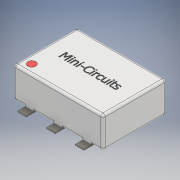
# Autodesk Inventor part: Transformer_CD542
Saved by Autodesk Inventor 2018 (Build 220112000, 112)
## iProperties
Created: 2019-01-11
Part Number: Transformer_CD542
Material: Copper
Document SubType Name: Modeling
Designer: Bradley
Density: 8.94 g/cm^3
Appearance: Smooth - White
Author: Bradley
Autodesk Inventor part; units mm, degrees
ref_plane "YZ Plane" through (0, 0, 0) normal (1, 0, 0) x (0, 1, 0)
ref_plane "XZ Plane" through (0, 0, 0) normal (0, 1, 0) x (-1, 0, 0)
ref_plane "XY Plane" through (0, 0, 0) normal (0, 0, 1) x (1, 0, 0)
sketch "Sketch1" plane through (0, 0, 0) normal (0, 0, 1) x (1, 0, 0)
  line L0 (-3.935, -2.795) -> (3.935, -2.795)
  line L1 (3.935, -2.795) -> (3.935, 2.795)
  line L2 (3.935, 2.795) -> (-3.935, 2.795)
  line L3 (-3.935, 2.795) -> (-3.935, -2.795)
  line L4 (-3.935, -2.795) -> (3.935, 2.795) construction
  line L5 (3.935, -2.795) -> (-3.935, 2.795) construction
  point P0 (0, 0)
  dimension "d0" = 7.87
  dimension "d1" = 5.59
  constraints: 12 end point, 2 midpoint, 2 parallel, 1 horizontal, 1 perpendicular
  measures "d0" distance of L2.end L1.end
  measures "d1" distance of L1.end L0.end
extrude "Extrusion1" add sketch "Sketch1" along normal blind 2.74
sketch "Sketch2" plane through (0, 0, 0) normal (0, 0, -1) x (-1, 0, 0)
  line L0 (3.935, -2.795) -> (-3.935, -2.795) projected
  line L1 (3.935, 2.795) -> (3.935, -2.795) projected
  line L2 (-3.935, 2.795) -> (3.935, 2.795) projected
  line L3 (-3.935, -2.795) -> (-3.935, 2.795) projected
  line L4 (-2.92, 3.455) -> (-2.16, 3.455)
  line L5 (-2.16, 3.455) -> (-2.16, 1.455)
  line L6 (-2.16, 1.455) -> (-2.92, 1.455)
  line L7 (-2.92, 1.455) -> (-2.92, 3.455)
  line L8 (-0.38, 3.455) -> (0.38, 3.455)
  line L9 (0.38, 3.455) -> (0.38, 1.455)
  line L10 (0.38, 1.455) -> (-0.38, 1.455)
  line L11 (-0.38, 1.455) -> (-0.38, 3.455)
  line L12 (2.16, 3.455) -> (2.92, 3.455)
  line L13 (2.92, 3.455) -> (2.92, 1.455)
  line L14 (2.92, 1.455) -> (2.16, 1.455)
  line L15 (2.16, 1.455) -> (2.16, 3.455)
  line L16 (-2.92, -1.455) -> (-2.16, -1.455)
  line L17 (-2.16, -1.455) -> (-2.16, -3.455)
  line L18 (-2.16, -3.455) -> (-2.92, -3.455)
  line L19 (-2.92, -3.455) -> (-2.92, -1.455)
  line L20 (-0.38, -1.455) -> (0.38, -1.455)
  line L21 (0.38, -1.455) -> (0.38, -3.455)
  line L22 (0.38, -3.455) -> (-0.38, -3.455)
  line L23 (-0.38, -3.455) -> (-0.38, -1.455)
  line L24 (2.16, -1.455) -> (2.92, -1.455)
  line L25 (2.92, -1.455) -> (2.92, -3.455)
  line L26 (2.92, -3.455) -> (2.16, -3.455)
  line L27 (2.16, -3.455) -> (2.16, -1.455)
  line L28 (-2.92, 1.455) -> (-2.92, -1.455) construction
  line L29 (-3.935, -2.795) -> (-3.935, 2.795) construction
  point P0 (0, 0)
  point P1 (0, 3.455)
  point P2 (-2.92, 0)
  dimension "d6" = 2.54
  dimension "d9" = 4.91
  dimension "d12" = 0.76
  dimension "d13" = 6.91
  dimension "d14" = 2
  constraints: 50 end point, 3 parallel, 2 horizontal, 2 midpoint, 1 horizontal alignment, 1 perpendicular, 1 vertical, 1 vertical alignment, 40 other
  measures "d6" distance of L4.start L8.start
  measures "d9" distance of L4.start L16.start
  measures "d12" distance of L5.end L6.end
  measures "d13" distance between parallel lines of L18 L4
  measures "d14" distance of L4.end L5.end
extrude "Extrusion2" add sketch "Sketch2" along normal blind 0.1 contours L25 L26 L27 L0 | L0 L27 L24 L25 | L13 L14 L15 L2 | L2 L15 L12 L13 | L21 L22 L23 L0 | L0 L23 L20 L21 | L9 L10 L11 L2 | L2 L11 L8 L9 | L17 L18 L19 L0 | L0 L19 L16 L17 | L5 L6 L7 L2 | L2 L7 L4 L5
fillet "Fillet1" radius 0.2 18 edges at (-3.935, 0, 0) (-3.935, -2.795, 1.37) (-3.935, 0, 2.74) (-3.935, 2.795, 1.37) (3.4275, 2.795, 0) (1.27, 2.795, 0) (-1.27, 2.795, 0) (-3.4275, 2.795, 0) (0, 2.795, 2.74) (3.935, 2.795, 1.37) (3.935, 0, 0) (3.935, 0, 2.74) (3.935, -2.795, 1.37) (-3.4275, -2.795, 0) (-1.27, -2.795, 0) (1.27, -2.795, 0) (3.4275, -2.795, 0) (0, -2.795, 2.74)
sketch "Sketch3" plane through (0, 0, 2.74) normal (0, 0, 1) x (1, 0, 0)
  line L0 (-3.735, -2.595) -> (-3.735, 2.595) projected
  line L1 (3.735, -2.595) -> (-3.735, -2.595) projected
  line L2 (3.735, 2.595) -> (3.735, -2.595) projected
  line L3 (-3.735, 2.595) -> (3.735, 2.595) projected
  circle A0 centre (-3.135, -1.995) radius 0.35
  circle A1 centre (-3.135, -1.995) radius 0.6 construction
  line L4 (-3.735, -2.595) -> (-3.735, 2.595) construction
  line L5 (-3.735, -0.2674) -> (3.735, -0.2674) construction
  line L6 (-1.912, -0.2674) -> (-2.005, -0.2674)
  line L7 (-2.005, -0.2674) -> (-2.005, 0.3356)
  line L8 (-2.005, 0.3356) -> (-2.1876, -0.0745)
  line L9 (-2.1876, -0.0745) -> (-2.2444, -0.0745)
  line L10 (-2.2444, -0.0745) -> (-2.4253, 0.3356)
  line L11 (-2.4253, 0.3356) -> (-2.4253, -0.2674)
  line L12 (-2.4253, -0.2674) -> (-2.5121, -0.2674)
  line L13 (-2.5121, -0.2674) -> (-2.5121, 0.4326)
  line L14 (-2.5121, 0.4326) -> (-2.385, 0.4326)
  line L15 (-2.385, 0.4326) -> (-2.2103, 0.0429)
  line L16 (-2.2103, 0.0429) -> (-2.0413, 0.4326)
  line L17 (-2.0413, 0.4326) -> (-1.912, 0.4326)
  line L18 (-1.912, 0.4326) -> (-1.912, -0.2674)
  line L19 (-1.6868, -0.2674) -> (-1.7752, -0.2674)
  line L20 (-1.7752, -0.2674) -> (-1.7752, 0.2579)
  line L21 (-1.7752, 0.2579) -> (-1.6868, 0.2579)
  line L22 (-1.6868, 0.2579) -> (-1.6868, -0.2674)
  line L23 (-1.6805, 0.3453) -> (-1.7809, 0.3453)
  line L24 (-1.7809, 0.3453) -> (-1.7809, 0.4372)
  line L25 (-1.7809, 0.4372) -> (-1.6805, 0.4372)
  line L26 (-1.6805, 0.4372) -> (-1.6805, 0.3453)
  line L27 (-1.1444, -0.2674) -> (-1.2329, -0.2674)
  line L28 (-1.2329, -0.2674) -> (-1.2329, 0.0322)
  spline S0 degree 2 poles (-1.2329, 0.0322) (-1.2329, 0.0685) (-1.2397, 0.1309) (-1.25, 0.1496) knots 0 0 0 1 2 2 2
  spline S1 degree 2 poles (-1.25, 0.1496) (-1.2607, 0.1694) (-1.2993, 0.1887) (-1.3322, 0.1887) knots 0 0 0 1 2 2 2
  spline S2 degree 2 poles (-1.3322, 0.1887) (-1.3651, 0.1887) (-1.4349, 0.1535) (-1.4684, 0.1252) knots 0 0 0 1 2 2 2
  line L29 (-1.4684, 0.1252) -> (-1.4684, -0.2674)
  line L30 (-1.4684, -0.2674) -> (-1.5568, -0.2674)
  line L31 (-1.5568, -0.2674) -> (-1.5568, 0.2579)
  line L32 (-1.5568, 0.2579) -> (-1.4684, 0.2579)
  line L33 (-1.4684, 0.2579) -> (-1.4684, 0.1995)
  spline S3 degree 2 poles (-1.4684, 0.1995) (-1.4286, 0.2352) (-1.3521, 0.2727) (-1.309, 0.2727) knots 0 0 0 1 2 2 2
  spline S4 degree 2 poles (-1.309, 0.2727) (-1.2318, 0.2727) (-1.1444, 0.1706) (-1.1444, 0.0736) knots 0 0 0 1 2 2 2
  line L34 (-1.1444, 0.0736) -> (-1.1444, -0.2674)
  line L35 (-0.93, -0.2674) -> (-1.0185, -0.2674)
  line L36 (-1.0185, -0.2674) -> (-1.0185, 0.2579)
  line L37 (-1.0185, 0.2579) -> (-0.93, 0.2579)
  line L38 (-0.93, 0.2579) -> (-0.93, -0.2674)
  line L39 (-0.9238, 0.3453) -> (-1.0242, 0.3453)
  line L40 (-1.0242, 0.3453) -> (-1.0242, 0.4372)
  line L41 (-1.0242, 0.4372) -> (-0.9238, 0.4372)
  line L42 (-0.9238, 0.4372) -> (-0.9238, 0.3453)
  line L43 (-0.5568, -0.0036) -> (-0.8217, -0.0036)
  line L44 (-0.8217, -0.0036) -> (-0.8217, 0.0815)
  line L45 (-0.8217, 0.0815) -> (-0.5568, 0.0815)
  line L46 (-0.5568, 0.0815) -> (-0.5568, -0.0036)
  spline S5 degree 2 poles (-0.1705, -0.2798) (-0.2385, -0.2798) (-0.3537, -0.2339) (-0.3957, -0.1879) knots 0 0 0 1 2 2 2
  spline S6 degree 2 poles (-0.3957, -0.1879) (-0.4376, -0.1426) (-0.4836, -0.0064) (-0.4836, 0.0821) knots 0 0 0 1 2 2 2
  spline S7 degree 2 poles (-0.4836, 0.0821) (-0.4836, 0.17) (-0.4388, 0.3005) (-0.3962, 0.3487) knots 0 0 0 1 2 2 2
  spline S8 degree 2 poles (-0.3962, 0.3487) (-0.3543, 0.3958) (-0.2397, 0.4451) (-0.1688, 0.4451) knots 0 0 0 1 2 2 2
  spline S9 degree 2 poles (-0.1688, 0.4451) (-0.1336, 0.4451) (-0.0718, 0.4349) (-0.0457, 0.427) knots 0 0 0 1 2 2 2
  spline S10 degree 2 poles (-0.0457, 0.427) (-0.023, 0.4196) (0.0241, 0.3986) (0.0474, 0.3861) knots 0 0 0 1 2 2 2
  line L47 (0.0474, 0.3861) -> (0.0474, 0.2738)
  line L48 (0.0474, 0.2738) -> (0.04, 0.2738)
  spline S11 degree 2 poles (0.04, 0.2738) (0.0275, 0.2852) (-0.0111, 0.3169) (-0.0389, 0.3322) knots 0 0 0 1 2 2 2
  spline S12 degree 2 poles (-0.0389, 0.3322) (-0.0655, 0.347) (-0.1285, 0.3657) (-0.1693, 0.3657) knots 0 0 0 1 2 2 2
  spline S13 degree 2 poles (-0.1693, 0.3657) (-0.2141, 0.3657) (-0.2941, 0.3288) (-0.3242, 0.2937) knots 0 0 0 1 2 2 2
  spline S14 degree 2 poles (-0.3242, 0.2937) (-0.3537, 0.2579) (-0.3866, 0.1496) (-0.3866, 0.0821) knots 0 0 0 1 2 2 2
  spline S15 degree 2 poles (-0.3866, 0.0821) (-0.3866, 0.01) (-0.352, -0.0938) (-0.3219, -0.1295) knots 0 0 0 1 2 2 2
  spline S16 degree 2 poles (-0.3219, -0.1295) (-0.2924, -0.1641) (-0.2136, -0.1993) (-0.1693, -0.1993) knots 0 0 0 1 2 2 2
  spline S17 degree 2 poles (-0.1693, -0.1993) (-0.1291, -0.1993) (-0.0604, -0.1794) (-0.0338, -0.1647) knots 0 0 0 1 2 2 2
  spline S18 degree 2 poles (-0.0338, -0.1647) (-0.0082, -0.1499) (0.0298, -0.1193) (0.0406, -0.1085) knots 0 0 0 1 2 2 2
  line L49 (0.0406, -0.1085) -> (0.0474, -0.1085)
  line L50 (0.0474, -0.1085) -> (0.0474, -0.2197)
  spline S19 degree 2 poles (0.0474, -0.2197) (0.0241, -0.2305) (-0.0167, -0.2503) (-0.0457, -0.2594) knots 0 0 0 1 2 2 2
  spline S20 degree 2 poles (-0.0457, -0.2594) (-0.0763, -0.2696) (-0.1285, -0.2798) (-0.1705, -0.2798) knots 0 0 0 1 2 2 2
  line L51 (0.2175, -0.2674) -> (0.1291, -0.2674)
  line L52 (0.1291, -0.2674) -> (0.1291, 0.2579)
  line L53 (0.1291, 0.2579) -> (0.2175, 0.2579)
  line L54 (0.2175, 0.2579) -> (0.2175, -0.2674)
  line L55 (0.2238, 0.3453) -> (0.1234, 0.3453)
  line L56 (0.1234, 0.3453) -> (0.1234, 0.4372)
  line L57 (0.1234, 0.4372) -> (0.2238, 0.4372)
  line L58 (0.2238, 0.4372) -> (0.2238, 0.3453)
  line L59 (0.626, 0.1632) -> (0.6214, 0.1632)
  spline S21 degree 2 poles (0.6214, 0.1632) (0.6112, 0.166) (0.5891, 0.1672) (0.5738, 0.1672) knots 0 0 0 1 2 2 2
  spline S22 degree 2 poles (0.5738, 0.1672) (0.538, 0.1672) (0.4677, 0.136) (0.4359, 0.1053) knots 0 0 0 1 2 2 2
  line L60 (0.4359, 0.1053) -> (0.4359, -0.2674)
  line L61 (0.4359, -0.2674) -> (0.3474, -0.2674)
  line L62 (0.3474, -0.2674) -> (0.3474, 0.2579)
  line L63 (0.3474, 0.2579) -> (0.4359, 0.2579)
  line L64 (0.4359, 0.2579) -> (0.4359, 0.1796)
  spline S23 degree 2 poles (0.4359, 0.1796) (0.4842, 0.2228) (0.5562, 0.2579) (0.5902, 0.2579) knots 0 0 0 1 2 2 2
  spline S24 degree 2 poles (0.5902, 0.2579) (0.6038, 0.2579) (0.6175, 0.2568) (0.626, 0.2551) knots 0 0 0 1 2 2 2
  line L65 (0.626, 0.2551) -> (0.626, 0.1632)
  spline S25 degree 2 poles (0.9034, -0.2793) (0.8489, -0.2793) (0.7587, -0.2458) (0.7264, -0.2118) knots 0 0 0 1 2 2 2
  spline S26 degree 2 poles (0.7264, -0.2118) (0.694, -0.1783) (0.6583, -0.0751) (0.6583, -0.0059) knots 0 0 0 1 2 2 2
  spline S27 degree 2 poles (0.6583, -0.0059) (0.6583, 0.0634) (0.6952, 0.1643) (0.7264, 0.1984) knots 0 0 0 1 2 2 2
  spline S28 degree 2 poles (0.7264, 0.1984) (0.7576, 0.233) (0.85, 0.2698) (0.9034, 0.2698) knots 0 0 0 1 2 2 2
  spline S29 degree 2 poles (0.9034, 0.2698) (0.9465, 0.2698) (1.027, 0.2454) (1.0582, 0.2296) knots 0 0 0 1 2 2 2
  line L66 (1.0582, 0.2296) -> (1.0582, 0.1303)
  line L67 (1.0582, 0.1303) -> (1.0531, 0.1303)
  spline S30 degree 2 poles (1.0531, 0.1303) (1.0435, 0.1382) (1.014, 0.1587) (0.993, 0.1694) knots 0 0 0 1 2 2 2
  spline S31 degree 2 poles (0.993, 0.1694) (0.9743, 0.1785) (0.9244, 0.1927) (0.9017, 0.1927) knots 0 0 0 1 2 2 2
  spline S32 degree 2 poles (0.9017, 0.1927) (0.833, 0.1927) (0.7496, 0.0889) (0.7496, -0.0059) knots 0 0 0 1 2 2 2
  spline S33 degree 2 poles (0.7496, -0.0059) (0.7496, -0.0983) (0.8302, -0.2021) (0.9017, -0.2021) knots 0 0 0 1 2 2 2
  spline S34 degree 2 poles (0.9017, -0.2021) (0.9448, -0.2021) (1.0231, -0.1664) (1.0531, -0.1386) knots 0 0 0 1 2 2 2
  line L68 (1.0531, -0.1386) -> (1.0582, -0.1386)
  line L69 (1.0582, -0.1386) -> (1.0582, -0.2379)
  spline S35 degree 2 poles (1.0582, -0.2379) (1.0452, -0.2441) (1.0055, -0.2617) (0.9896, -0.2657) knots 0 0 0 1 2 2 2
  spline S36 degree 2 poles (0.9896, -0.2657) (0.9669, -0.2725) (0.9312, -0.2793) (0.9034, -0.2793) knots 0 0 0 1 2 2 2
  line L70 (1.5472, -0.2674) -> (1.4587, -0.2674)
  line L71 (1.4587, -0.2674) -> (1.4587, -0.2095)
  spline S37 degree 2 poles (1.4587, -0.2095) (1.4179, -0.2452) (1.3447, -0.2821) (1.2993, -0.2821) knots 0 0 0 1 2 2 2
  spline S38 degree 2 poles (1.2993, -0.2821) (1.2653, -0.2821) (1.2046, -0.2594) (1.1825, -0.235) knots 0 0 0 1 2 2 2
  spline S39 degree 2 poles (1.1825, -0.235) (1.1598, -0.2106) (1.1348, -0.1363) (1.1348, -0.083) knots 0 0 0 1 2 2 2
  line L72 (1.1348, -0.083) -> (1.1348, 0.2579)
  line L73 (1.1348, 0.2579) -> (1.2233, 0.2579)
  line L74 (1.2233, 0.2579) -> (1.2233, -0.0416)
  spline S40 degree 2 poles (1.2233, -0.0416) (1.2233, -0.0836) (1.2295, -0.1386) (1.2403, -0.159) knots 0 0 0 1 2 2 2
  spline S41 degree 2 poles (1.2403, -0.159) (1.2511, -0.1794) (1.288, -0.1982) (1.3226, -0.1982) knots 0 0 0 1 2 2 2
  spline S42 degree 2 poles (1.3226, -0.1982) (1.3549, -0.1982) (1.4281, -0.1613) (1.4587, -0.1346) knots 0 0 0 1 2 2 2
  line L75 (1.4587, -0.1346) -> (1.4587, 0.2579)
  line L76 (1.4587, 0.2579) -> (1.5472, 0.2579)
  line L77 (1.5472, 0.2579) -> (1.5472, -0.2674)
  line L78 (1.7656, -0.2674) -> (1.6771, -0.2674)
  line L79 (1.6771, -0.2674) -> (1.6771, 0.2579)
  line L80 (1.6771, 0.2579) -> (1.7656, 0.2579)
  line L81 (1.7656, 0.2579) -> (1.7656, -0.2674)
  line L82 (1.7718, 0.3453) -> (1.6714, 0.3453)
  line L83 (1.6714, 0.3453) -> (1.6714, 0.4372)
  line L84 (1.6714, 0.4372) -> (1.7718, 0.4372)
  line L85 (1.7718, 0.4372) -> (1.7718, 0.3453)
  spline S43 degree 2 poles (2.0543, -0.2776) (1.9823, -0.2776) (1.9012, -0.1953) (1.9012, -0.1063) knots 0 0 0 1 2 2 2
  line L86 (1.9012, -0.1063) -> (1.9012, 0.1847)
  line L87 (1.9012, 0.1847) -> (1.8416, 0.1847)
  line L88 (1.8416, 0.1847) -> (1.8416, 0.2579)
  line L89 (1.8416, 0.2579) -> (1.9012, 0.2579)
  line L90 (1.9012, 0.2579) -> (1.9012, 0.4088)
  line L91 (1.9012, 0.4088) -> (1.9897, 0.4088)
  line L92 (1.9897, 0.4088) -> (1.9897, 0.2579)
  line L93 (1.9897, 0.2579) -> (2.1525, 0.2579)
  line L94 (2.1525, 0.2579) -> (2.1525, 0.1847)
  line L95 (2.1525, 0.1847) -> (1.9897, 0.1847)
  line L96 (1.9897, 0.1847) -> (1.9897, -0.0654)
  spline S44 degree 2 poles (1.9897, -0.0654) (1.9897, -0.1051) (1.9925, -0.1488) (2.0021, -0.1675) knots 0 0 0 1 2 2 2
  spline S45 degree 2 poles (2.0021, -0.1675) (2.0101, -0.184) (2.0458, -0.2004) (2.0765, -0.2004) knots 0 0 0 1 2 2 2
  spline S46 degree 2 poles (2.0765, -0.2004) (2.098, -0.2004) (2.1383, -0.1874) (2.1474, -0.1834) knots 0 0 0 1 2 2 2
  line L97 (2.1474, -0.1834) -> (2.1525, -0.1834)
  line L98 (2.1525, -0.1834) -> (2.1525, -0.2628)
  spline S47 degree 2 poles (2.1525, -0.2628) (2.1275, -0.2696) (2.0765, -0.2776) (2.0543, -0.2776) knots 0 0 0 1 2 2 2
  spline S48 degree 2 poles (2.3595, -0.2798) (2.3068, -0.2798) (2.2154, -0.2515) (2.1854, -0.2356) knots 0 0 0 1 2 2 2
  line L99 (2.1854, -0.2356) -> (2.1854, -0.1363)
  line L100 (2.1854, -0.1363) -> (2.1899, -0.1363)
  spline S49 degree 2 poles (2.1899, -0.1363) (2.2013, -0.1454) (2.2319, -0.167) (2.2574, -0.1789) knots 0 0 0 1 2 2 2
  spline S50 degree 2 poles (2.2574, -0.1789) (2.2795, -0.1896) (2.334, -0.2055) (2.3629, -0.2055) knots 0 0 0 1 2 2 2
  spline S51 degree 2 poles (2.3629, -0.2055) (2.3839, -0.2055) (2.4321, -0.1959) (2.4435, -0.1879) knots 0 0 0 1 2 2 2
  spline S52 degree 2 poles (2.4435, -0.1879) (2.4599, -0.1772) (2.4747, -0.1528) (2.4747, -0.1278) knots 0 0 0 1 2 2 2
  spline S53 degree 2 poles (2.4747, -0.1278) (2.4747, -0.0966) (2.4406, -0.0643) (2.397, -0.0535) knots 0 0 0 1 2 2 2
  spline S54 degree 2 poles (2.397, -0.0535) (2.3799, -0.0495) (2.3255, -0.0382) (2.3022, -0.0319) knots 0 0 0 1 2 2 2
  spline S55 degree 2 poles (2.3022, -0.0319) (2.2421, -0.0144) (2.1876, 0.0582) (2.1876, 0.1099) knots 0 0 0 1 2 2 2
  spline S56 degree 2 poles (2.1876, 0.1099) (2.1876, 0.1813) (2.2949, 0.2704) (2.3833, 0.2704) knots 0 0 0 1 2 2 2
  spline S57 degree 2 poles (2.3833, 0.2704) (2.427, 0.2704) (2.5155, 0.2488) (2.5456, 0.2324) knots 0 0 0 1 2 2 2
  line L101 (2.5456, 0.2324) -> (2.5456, 0.1377)
  line L102 (2.5456, 0.1377) -> (2.541, 0.1377)
  spline S58 degree 2 poles (2.541, 0.1377) (2.507, 0.1649) (2.4242, 0.1961) (2.3816, 0.1961) knots 0 0 0 1 2 2 2
  spline S59 degree 2 poles (2.3816, 0.1961) (2.338, 0.1961) (2.2778, 0.1592) (2.2778, 0.1223) knots 0 0 0 1 2 2 2
  spline S60 degree 2 poles (2.2778, 0.1223) (2.2778, 0.0889) (2.3136, 0.0565) (2.3533, 0.0463) knots 0 0 0 1 2 2 2
  spline S61 degree 2 poles (2.3533, 0.0463) (2.3726, 0.0412) (2.4214, 0.031) (2.448, 0.0248) knots 0 0 0 1 2 2 2
  spline S62 degree 2 poles (2.448, 0.0248) (2.5059, 0.01) (2.5649, -0.0575) (2.5649, -0.1159) knots 0 0 0 1 2 2 2
  spline S63 degree 2 poles (2.5649, -0.1159) (2.5649, -0.1499) (2.5382, -0.2101) (2.5121, -0.2322) knots 0 0 0 1 2 2 2
  spline S64 degree 2 poles (2.5121, -0.2322) (2.4843, -0.2554) (2.4134, -0.2798) (2.3595, -0.2798) knots 0 0 0 1 2 2 2
  point P0 (0, 0)
  dimension "d18" = 0.7
  dimension "d19" = 1.2
  constraints: 2 centre point, 2 end point, 2 point on line, 2 tangent, 1 coincident, 1 horizontal, 1 perpendicular
  measures "d18" diameter of A0
  measures "d19" diameter of A1
extrude "Extrusion3" add sketch "Sketch3" along normal blind 0.01 contours A0
extrude "Extrusion4" add sketch "Sketch3" along normal blind 0.01 contours L6 L7 L8 L9 L10 L11 L12 L13 L14 L15 L16 L17 L18 | L19 L20 L21 L22 | L23 L24 L25 L26 | L27 L28 S0 S1 S2 L29 L30 L31 L32 L33 S3 S4 L34 | L35 L36 L37 L38 | L39 L40 L41 L42 | L43 L44 L45 L46 | S5 S6 S7 S8 S9 S10 L47 L48 S11 S12 S13 S14 S15 S16 S17 S18 L49 L50 S19 S20 | L51 L52 L53 L54 | L55 L56 L57 L58 | L59 S21 S22 L60 L61 L62 L63 L64 S23 S24 L65 | S25 S26 S27 S28 S29 L66 L67 S30 S31 S32 S33 S34 L68 L69 S35 S36 | L70 L71 S37 S38 S39 L72 L73 L74 S40 S41 S42 L75 L76 L77 | L78 L79 L80 L81 | L82 L83 L84 L85 | S43 L86 L87 L88 L89 L90 L91 L92 L93 L94 L95 L96 S44 S45 S46 L97 L98 S47 | S48 L99 L100 S49 S50 S51 S52 S53 S54 S55 S56 S57 L101 L102 S58 S59 S60 S61 S62 S63 S64
body "Solid1"
